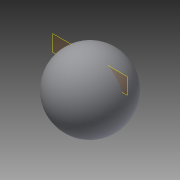
# Autodesk Inventor part: Ball
Saved by Autodesk Inventor 2013 (Build 170138000, 138)
## iProperties
Created: 2014-01-09
Part Number: Ball
Material: Generic
Document SubType Name: Modeling
Designer: 215152
Density: 1 g/cm^3
Author: 215152
Autodesk Inventor part; units mm, degrees
ref_plane "YZ Plane" through (0, 0, 0) normal (1, 0, 0) x (0, 1, 0)
ref_plane "XZ Plane" through (0, 0, 0) normal (0, 1, 0) x (-1, 0, 0)
ref_plane "XY Plane" through (0, 0, 0) normal (0, 0, 1) x (1, 0, 0)
ref_plane "Work Plane1" through (0, 0, 304.8) normal (0, 0, 1) x (1, 0, 0)
sketch "Sketch1" plane through (0, 0, 304.8) normal (0, 0, 1) x (1, 0, 0)
  line L0 (0, 0) -> (0, 114.3)
  line L1 (0, 114.3) -> (0, -190.5)
  circle A0 centre (0, -190.5) radius 304.8
  line L2 (-304.7246, -183.7194) -> (304.7246, -197.2806)
  dimension "d0" = 114.3
  dimension "d1" = 304.8
  dimension "d2" = 0
  dimension "d3" = 609.6
  constraints: 6 end point, 2 point on circle, 1 centre point, 1 coincident, 1 collinear, 1 midpoint, 1 vertical
  measures "d0" distance of L0.start L0.end
  measures "d1" distance of L0.end L1.end
  measures "d2" distance between parallel lines of L1 L0
  measures "d3" diameter of A0
revolve "Revolution1" add sketch "Sketch1" angle 360 about axis through (-304.7246, -183.7194, 304.8) along (0.9997525, -0.022246, 0) contours L2 A0
body "Solid1"
